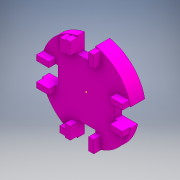
# Autodesk Inventor part: Circuit
Saved by Autodesk Inventor 2018 (Build 220112000, 112)
## iProperties
Created: 2018-01-14
Part Number: Circuit
Material: Generic
Document SubType Name: Modeling
Designer: Suchanek
Density: 1 g/cm^3
Appearance: Default
Author: Suchanek
Autodesk Inventor part; units mm, degrees
ref_plane "YZ Plane" through (0, 0, 0) normal (1, 0, 0) x (0, 1, 0)
ref_plane "XZ Plane" through (0, 0, 0) normal (0, 1, 0) x (-1, 0, 0)
ref_plane "XY Plane" through (0, 0, 0) normal (0, 0, 1) x (1, 0, 0)
sketch "Sketch4" plane through (0, 0, 0) normal (0, 1, 0) x (-1, 0, 0)
  circle A0 centre (0, 0) radius 32
  dimension "d48" = 64
  constraints: 1 centre point, 1 coincident
  measures "d48" diameter of A0
extrude "Extrusion1" add sketch "Sketch4" along normal blind 5
sketch "Sketch5" plane through (0, 5, 0) normal (0, 1, 0) x (1, 0, 0)
  line L0 (-6.5, -32) -> (6.5, -32)
  line L1 (6.5, -32) -> (6.5, -20)
  line L2 (6.5, -20) -> (-6.5, -20)
  line L3 (-6.5, -20) -> (-6.5, -32)
  line L4 (-32, -6.5) -> (-20, -6.5)
  line L5 (-20, -6.5) -> (-20, 6.5)
  line L6 (-20, 6.5) -> (-32, 6.5)
  line L7 (-32, 6.5) -> (-32, -6.5)
  line L8 (-6.5, 20) -> (6.5, 20)
  line L9 (6.5, 20) -> (6.5, 32)
  line L10 (6.5, 32) -> (-6.5, 32)
  line L11 (-6.5, 32) -> (-6.5, 20)
  line L12 (20, -6.5) -> (32, -6.5)
  line L13 (32, -6.5) -> (32, 6.5)
  line L14 (32, 6.5) -> (20, 6.5)
  line L15 (20, 6.5) -> (20, -6.5)
  line L16 (0, 0) -> (-6.9492, 0)
  line L17 (0, 0) -> (0, 8.4834)
  dimension "d51" = 13
  dimension "d52" = 12
  dimension "d53" = 12
  dimension "d54" = 13
  dimension "d57" = 13
  dimension "d58" = 12
  dimension "d59" = 12
  dimension "d60" = 13
  dimension "d61" = 40
  dimension "d62" = 40
  constraints: 36 end point, 8 parallel, 5 horizontal, 4 perpendicular, 2 collinear, 1 vertical, 4 other
  measures "d51" distance of L2.end L1.end
  measures "d52" distance of L1.end L0.end
  measures "d53" distance of L6.end L5.end
  measures "d54" distance of L5.end L4.end
  measures "d57" distance of L10.end L9.end
  measures "d58" distance of L9.end L8.end
  measures "d59" distance of L14.end L13.end
  measures "d60" distance of L13.end L12.end
  measures "d61" distance between parallel lines of L15 L5
  measures "d62" distance between parallel lines of L8 L2
extrude "Extrusion2" cut sketch "Sketch5" against normal blind 5
sketch "Sketch6" plane through (0, 5, 0) normal (0, 1, 0) x (1, 0, 0)
  arc A0 (6.5, -31.3329) -> (31.3329, -6.5) centre (0, 0) ccw projected
  line L0 (31.3329, -6.5) -> (6.5, -6.5)
  line L1 (6.5, -6.5) -> (6.5, -31.3329)
  line L2 (6.5, -31.3329) -> (6.5, -20) projected
  arc A1 (6.5, -31.3329) -> (31.3329, -6.5) centre (0, 0) ccw
  constraints: 4 end point, 2 point on circle, 1 centre point, 1 coincident
extrude "Extrusion3" add sketch "Sketch6" along normal blind 5
sketch "Sketch7" plane through (0, 5, 0) normal (0, 1, 0) x (1, 0, 0)
  line L0 (-20, 6.5) -> (-20, -6.5) projected
  line L1 (-20, 6.5) -> (-20, 20)
  line L2 (6.5, 20) -> (-6.5, 20) projected
  line L3 (-6.5, 20) -> (-20, 20)
  line L4 (-20, 18.5) -> (-13.5, 18.5)
  line L5 (-13.5, 18.5) -> (-13.5, 15.5)
  line L6 (-13.5, 15.5) -> (-20, 15.5)
  line L7 (-20, 15.5) -> (-20, 18.5)
  line L8 (-6.5, 20) -> (-6.5, 31.3329) projected
  point P0 (0, 0)
  dimension "d69" = 7
  dimension "d70" = 1.5
  dimension "d71" = 6.5
  dimension "d72" = 3
  constraints: 12 end point, 2 parallel, 1 collinear, 1 horizontal, 1 perpendicular, 1 point on line, 1 vertical
  measures "d69" distance between parallel lines of L5 L8
  measures "d70" distance between parallel lines of L3 L4
  measures "d71" distance between parallel lines of L1 L5
  measures "d72" distance between parallel lines of L6 L4
extrude "Extrusion4" add sketch "Sketch7" along normal blind 5
sketch "Sketch8" plane through (0, 0, 0) normal (0, -1, 0) x (1, 0, 0)
  point P0 (0, 0)
sketch "Sketch9" plane through (0, 0, 0) normal (0, -1, 0) x (1, 0, 0)
  line L0 (-31.3329, -6.5) -> (-20, -6.5) projected
  line L1 (-30.4, -6.5) -> (-21.7, -6.5)
  line L2 (-21.7, -6.5) -> (-21.7, -10.2)
  line L3 (-21.7, -10.2) -> (-30.4, -10.2)
  line L4 (-30.4, -10.2) -> (-30.4, -6.5)
  line L5 (-20, 6.5) -> (-31.3329, 6.5) projected
  line L6 (-21.7, 6.5) -> (-30.4, 6.5)
  line L7 (-30.4, 6.5) -> (-30.4, 10.2)
  line L8 (-30.4, 10.2) -> (-21.7, 10.2)
  line L9 (-21.7, 10.2) -> (-21.7, 6.5)
  line L10 (6.5, 31.3329) -> (6.5, 20) projected
  line L11 (6.5, 21.7) -> (10.2, 21.7)
  line L12 (10.2, 21.7) -> (10.2, 30.4)
  line L13 (10.2, 30.4) -> (6.5, 30.4)
  line L14 (6.5, 30.4) -> (6.5, 21.7)
  line L15 (6.5, -31.3329) -> (6.5, -20) projected
  line L16 (6.5, -21.7) -> (10.2, -21.7)
  line L17 (10.2, -21.7) -> (10.2, -30.4)
  line L18 (10.2, -30.4) -> (6.5, -30.4)
  line L19 (6.5, -30.4) -> (6.5, -21.7)
  line L20 (20, 6.5) -> (31.3329, 6.5) projected
  line L21 (21.7, 6.5) -> (30.4, 6.5)
  line L22 (30.4, 6.5) -> (30.4, 10.2)
  line L23 (30.4, 10.2) -> (21.7, 10.2)
  line L24 (21.7, 10.2) -> (21.7, 6.5)
  line L25 (21.7, -6.5) -> (30.4, -6.5)
  line L26 (30.4, -6.5) -> (30.4, -10.2)
  line L27 (30.4, -10.2) -> (21.7, -10.2)
  line L28 (21.7, -10.2) -> (21.7, -6.5)
  line L29 (-6.5, -20) -> (-6.5, -31.3329) projected
  line L30 (-6.5, -30.4) -> (-10.2, -30.4)
  line L31 (-10.2, -30.4) -> (-10.2, -21.7)
  line L32 (-10.2, -21.7) -> (-6.5, -21.7)
  line L33 (-6.5, -21.7) -> (-6.5, -30.4)
  line L34 (-6.5, 31.3329) -> (-6.5, 20) projected
  line L35 (-10.2, 21.4) -> (-6.5, 21.4)
  line L36 (-6.5, 21.4) -> (-6.5, 30.1)
  line L37 (-6.5, 30.1) -> (-10.2, 30.1)
  line L38 (-10.2, 30.1) -> (-10.2, 21.4)
  line L39 (-6.5, -20) -> (6.5, -20) projected
  line L40 (20, -6.5) -> (20, 6.5) projected
  line L41 (6.5, 20) -> (-6.5, 20) projected
  line L42 (-20, 6.5) -> (-20, -6.5) projected
  line L43 (-10.2, -29.4) -> (-13.9, -29.4)
  line L44 (-13.9, -29.4) -> (-13.9, -25.1)
  line L45 (-13.9, -25.1) -> (-10.2, -25.1)
  line L46 (-10.2, -25.1) -> (-10.2, -29.4)
  line L47 (-13.9, 20.4) -> (-10.2, 20.4)
  line L48 (-10.2, 20.4) -> (-10.2, 29.1)
  line L49 (-10.2, 29.1) -> (-13.9, 29.1)
  line L50 (-13.9, 29.1) -> (-13.9, 20.4)
  point P0 (0, 0)
  dimension "d75" = 1.7
  dimension "d76" = 8.7
  dimension "d77" = 3.7
  dimension "d78" = 1.7
  dimension "d79" = 8.7
  dimension "d80" = 3.7
  dimension "d81" = 1.7
  dimension "d82" = 3.7
  dimension "d83" = 8.7
  dimension "d84" = 3.7
  dimension "d85" = 8.7
  dimension "d86" = 8.7
  dimension "d87" = 1.7
  dimension "d90" = 1.7
  dimension "d91" = 8.7
  dimension "d96" = 3.7
  dimension "d97" = 4.3
  dimension "d98" = 1
  dimension "d101" = 10.1
  dimension "d102" = 3.7
  dimension "d103" = 8.7
  dimension "d104" = 1
  constraints: 80 end point, 20 parallel, 17 point on line, 10 horizontal, 10 perpendicular, 1 collinear
  measures "d75" distance between parallel lines of L39 L32
  measures "d76" distance between parallel lines of L30 L32
  measures "d77" distance between parallel lines of L33 L31
  measures "d78" distance between parallel lines of L39 L16
  measures "d79" distance between parallel lines of L16 L18
  measures "d80" distance between parallel lines of L15 L17
  measures "d81" distance between parallel lines of L28 L40
  measures "d82" distance between parallel lines of L25 L27
  measures "d83" distance between parallel lines of L26 L28
  measures "d84" distance between parallel lines of L23 L20
  measures "d85" distance between parallel lines of L37 L35
  measures "d86" distance between parallel lines of L13 L11
  measures "d87" distance between parallel lines of L11 L41
  measures "d90" distance between parallel lines of L42 L9
  measures "d91" distance between parallel lines of L4 L2
  measures "d96" distance of L44.end L45.end
  measures "d97" distance of L43.end L44.end
  measures "d98" distance between parallel lines of L30 L43
  measures "d101" distance between parallel lines of L37 L41
  measures "d102" distance between parallel lines of L38 L50
  measures "d103" distance between parallel lines of L49 L47
  measures "d104" distance between parallel lines of L37 L49
extrude "Extrusion5" add sketch "Sketch9" along normal blind 5
body "Solid1"
